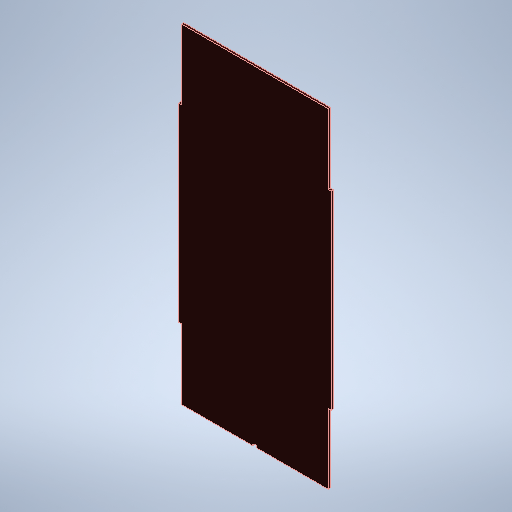
# Autodesk Inventor part: Finishing Sheets .3  ( Back )
Saved by Autodesk Inventor 2025.4 (Build 294407000, 407)
## iProperties
Created: 2026-04-04
Part Number: Finishing Sheets .3  ( Back )
Material: Generic
Document SubType Name: Sheet Metal
Designer: lenovo
Density: 1 g/cm^3
Sheet Metal Rule: Default_mm
Appearance: Default(2)
Author: lenovo
Autodesk Inventor part; units mm, degrees
ref_plane "YZ Plane" through (0, 0, 0) normal (1, 0, 0) x (0, 1, 0)
ref_plane "XZ Plane" through (0, 0, 0) normal (0, 1, 0) x (-1, 0, 0)
ref_plane "XY Plane" through (0, 0, 0) normal (0, 0, 1) x (1, 0, 0)
sketch "Sketch1" plane through (0, 0, 0) normal (0, 0, 1) x (1, 0, 0)
  line L0 (-96.5, -217) -> (96.5, -217)
  line L1 (96.5, -217) -> (96.5, 217)
  line L2 (-96.5, 217) -> (-96.5, -217)
  line L3 (-96.5, -217) -> (96.5, 217) construction
  line L4 (96.5, -217) -> (-96.5, 217) construction
  line L5 (-96.5, 217) -> (96.5, 217)
  line L6 (-96.5, 125) -> (-100.5, 125)
  line L7 (-100.5, 125) -> (-100.5, -125)
  line L8 (-100.5, -125) -> (-96.5, -125)
  line L9 (-96.5, -125) -> (-96.5, 125)
  line L10 (0, 217) -> (0, 0)
  line L11 (96.5, 125) -> (100.5, 125)
  line L12 (100.5, 125) -> (100.5, -125)
  line L13 (100.5, -125) -> (96.5, -125)
  line L14 (96.5, -125) -> (96.5, 125)
  point P0 (-100.5, 0)
  point P1 (-96.5, 0)
  point P2 (-96.5, -125)
  point P3 (100.5, 0)
  point P4 (96.5, 0)
  point P5 (96.5, 125)
  point P6 (96.5, -125)
  dimension "d0" = 434
  dimension "d1" = 193
  dimension "d3" = 4
  dimension "d4" = 250
  measures "d0" distance of L0.end L1.end
  measures "d1" distance of L0.start L0.end
  measures "d3" distance of L6.start L6.end
  measures "d4" distance of L6.end L7.end
extrude "Plate1" add sketch "Sketch1" along normal blind 3
sketch "Sketch2" plane through (0, 0, 3) normal (0, 0, 1) x (1, 0, 0)
  line L0 (-96.5, -217) -> (96.5, -217) projected
  arc A0 (3, -217) -> (-3, -217) centre (0, -217) ccw
  line L1 (96.5, -217) -> (-96.5, -217) projected
  point P0 (0, 0)
  dimension "d6" = 3
  constraints: 3 midpoint, 2 point on circle, 2 point on line, 1 centre point
  measures "d6" radius of A0
extrude "Cut1" cut sketch "Sketch2" against normal blind 3
equation "\"d7\" = Thickness"
equation "\"d5\" = Thickness"
equation "\"BendRadius\" = Thickness"
equation "\"BendReliefWidth\" = Thickness"
equation "\"BendReliefDepth\" = 0.5 * Thickness"
equation "\"CornerReliefSize\" = 4 * Thickness"
equation "\"MinimumRemnant\" = 2 * Thickness"
equation "\"TransitionRadius\" = BendRadius"
equation "\"JacobiRadiusSize\" = BendRadius"
equation "\"GapSize\" = Thickness"
equation "\"Thickness\" = 3"
body "Solid1"
